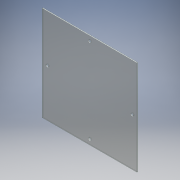
# Autodesk Inventor part: short covering
Saved by Autodesk Inventor 2016 (Build 200138000, 138)
## iProperties
Created: 2016-08-02
Part Number: short covering
Material: Glass
Document SubType Name: Modeling
Designer: Jonathan
Density: 2.18 g/cm^3
Appearance: Clear
Author: Jonathan
Autodesk Inventor part; units mm, degrees
ref_plane "YZ Plane" through (0, 0, 0) normal (1, 0, 0) x (0, 1, 0)
ref_plane "XZ Plane" through (0, 0, 0) normal (0, 1, 0) x (-1, 0, 0)
ref_plane "XY Plane" through (0, 0, 0) normal (0, 0, 1) x (1, 0, 0)
sketch "Sketch1" plane through (0, 0, 0) normal (0, 1, 0) x (-1, 0, 0)
  line L0 (95, -95) -> (-95, -95)
  line L1 (-95, -95) -> (-95, 95)
  line L2 (-95, 95) -> (95, 95)
  line L3 (95, 95) -> (95, -95)
  line L4 (95, -95) -> (-95, 95) construction
  line L5 (-95, -95) -> (95, 95) construction
  point P0 (0, 0)
  dimension "d0" = 190
  constraints: 12 end point, 2 midpoint, 2 parallel, 2 perpendicular, 1 horizontal
  measures "d0" distance of L0.start L0.end
extrude "Extrusion1" add sketch "Sketch1" along normal blind 1.5875
sketch "Sketch2" plane through (0, 1.5875, 0) normal (0, 1, 0) x (1, 0, 0)
  line L0 (-95, 95) -> (-95, -95) projected
  line L1 (-95, -95) -> (95, -95) projected
  line L2 (95, 95) -> (-95, 95) projected
  line L3 (-95, 95) -> (-95, -95) projected
  line L4 (-95, -95) -> (95, -95) projected
  line L5 (95, -95) -> (95, 95) projected
  point P0 (-85, 0)
  point P1 (0, -85)
  point P2 (85, 0)
  point P3 (0, 85)
  point P4 (0, 0)
  dimension "d17" = 10
  dimension "d18" = 10
  dimension "d19" = 10
  dimension "d20" = 10
  constraints: 2 horizontal alignment, 2 vertical alignment
  measures "d17" distance from line of L0 point (-85, 0)
  measures "d18" distance from line of L1 point (0, -85)
  measures "d19" distance from line of L5 point (85, 0)
  measures "d20" distance from line of L2 point (0, 85)
hole "Hole1" at (-85, 1.5875, 0) at (0, 1.5875, 85) at (85, 1.5875, 0) at (0, 1.5875, -85) direction (0, -1, 0) diameter 5.5 end through all clearance for "Flat Head Machine Screw" size "M5" standard "Ansi Metric M Profile"
body "Solid1"
